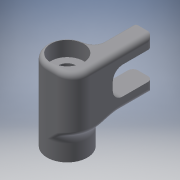
# Autodesk Inventor part: guia.tractora0.2
Saved by Autodesk Inventor 2016 (Build 200138000, 138)
## iProperties
Created: 2015-07-01
Part Number: guia.tractora0.2
Material: Generic
Document SubType Name: Modeling
Designer: pc
Density: 1 g/cm^3
Appearance: Default
Author: pc
Autodesk Inventor part; units mm, degrees
ref_plane "YZ Plane" through (0, 0, 0) normal (1, 0, 0) x (0, 1, 0)
ref_plane "XZ Plane" through (0, 0, 0) normal (0, 1, 0) x (-1, 0, 0)
ref_plane "XY Plane" through (0, 0, 0) normal (0, 0, 1) x (1, 0, 0)
sketch "Sketch10" plane through (0, 0, 0) normal (0, 0, 1) x (1, 0, 0)
  arc A0 (1.25, 3.799671) -> (0, -4) centre (0, 0) ccw
  line L0 (1.25, 3.799671) -> (1.25, 11.799671)
  line L1 (1.25, 11.799671) -> (5.25, 11.799671)
  line L2 (5.25, 11.799671) -> (5.25, -4)
  line L3 (5.25, -4) -> (0, -4)
  point P0 (1.25, -4)
  point P1 (1.25, -3)
  point P2 (3.25, 11.799671)
  dimension "d51" = 8
  dimension "d52" = 8
  dimension "d53" = 4
  dimension "d56" = 1.25
  constraints: 8 end point, 3 point on line, 2 perpendicular, 2 point on circle, 1 centre point, 1 coincident, 1 midpoint, 1 parallel, 1 tangent, 1 vertical
  measures "d51" diameter of A0
  measures "d52" distance of L0.start L0.end
  measures "d53" distance of L0.end L1.end
  measures "d56" distance from line of L0 point (0, 0)
extrude "Extrusion7" add sketch "Sketch10" along normal blind 10
sketch "Sketch15" plane through (0, 0, 0) normal (0, 0, -1) x (-1, 0, 0)
  arc A0 (0, -4) -> (-1.25, 3.799671) centre (0, 0) ccw
  circle A1 centre (0, 0) radius 4
  constraints: 1 centre point, 1 coincident, 1 concentric
extrude "Extrusion12" add sketch "Sketch15" along normal blind 6
sketch "Sketch16" plane through (0, 0, 10) normal (0, 0, 1) x (1, 0, 0)
  arc A0 (1.25, 3.799671) -> (0, -4) centre (0, 0) ccw
  circle A1 centre (0, 0) radius 3.25
  dimension "d71" = 6.5
  constraints: 1 centre point, 1 coincident
  measures "d71" diameter of A1
extrude "Extrusion13" cut sketch "Sketch16" against normal blind 3
sketch "Sketch17" plane through (0, 0, 7) normal (0, 0, 1) x (1, 0, 0)
  circle A0 centre (0, 0) radius 3.25 projected
  circle A1 centre (0, 0) radius 1.75
  dimension "d74" = 3.5
  constraints: 1 centre point, 1 coincident
  measures "d74" diameter of A1
extrude "Extrusion14" cut sketch "Sketch17" against normal through all contours A1
sketch "Sketch18" plane through (1.25, 3.799671, 0) normal (-1, 0, 0) x (0, 0, 1)
  line L0 (0, 8) -> (0, 0)
  line L1 (0, 0) -> (10, 0)
  line L2 (10, 8) -> (10, 0)
  line L3 (0, 8) -> (10, 8)
  line L4 (3.75, 2) -> (6.25, 2) construction
  line L5 (2.25, 8) -> (2.25, 0)
  line L6 (7.75, 8) -> (7.75, 0)
  point P0 (0, -3.799671)
  point P1 (7.75, 0.5)
  point P2 (5, 2)
  dimension "d79" = 6
  dimension "d80" = 5
  constraints: 16 end point, 5 point on line, 2 vertical, 1 horizontal, 1 midpoint
  measures "d79" distance from line of L3 point (5, 2)
  measures "d80" distance from line of L0 point (5, 2)
extrude "Extrusion16" cut sketch "Sketch18" against normal through all contours L3 L6 L1 L5
fillet "Fillet14" radius 2 3 edges at (3.25, 3.7997, 7.75) (3.25, 3.7997, 2.25) (1.25, 3.7997, 5)
fillet "Fillet5" radius 2.76 1 edges at (3.9921, 0.2505, 0)
fillet "Fillet9" radius 3.26 1 edges at (5.25, -4, 4.9977)
fillet "Fillet10" radius 1 16 edges at (5.25, 5.5298, 10) (4.2952, -3.0452, 10) (0.995, -4, 10) (-3.9921, -0.2505, 10) (1.25, 8.8763, 10) (1.25, 11.7997, 8.875) (1.25, 11.7997, 1.125) (1.25, 9.2215, 0) (1.25, 6.2956, -0.0212) (5.25, 8.0291, 0) (5.25, 1.7733, -0.2836) (4.2009, -3.1357, -0.4548) (1.6157, -4, -1.4815) (0.6194, -4, -2.2492) (5.25, 11.7997, 8.875) (5.25, 11.7997, 1.125)
body "Solid3"
